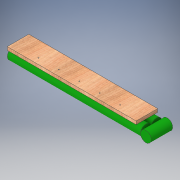
# Autodesk Inventor part: Bumper Side
Saved by Autodesk Inventor 2018 (Build 220112000, 112)
## iProperties
Created: 2019-02-24
Part Number: Bumper Side
Material: Generic
Document SubType Name: Modeling
Designer: maste
Density: 1 g/cm^3
Appearance: Default
Author: maste
Autodesk Inventor part; units mm, degrees
ref_plane "YZ Plane" through (0, 0, 0) normal (1, 0, 0) x (0, 1, 0)
ref_plane "XZ Plane" through (0, 0, 0) normal (0, 1, 0) x (-1, 0, 0)
ref_plane "XY Plane" through (0, 0, 0) normal (0, 0, 1) x (1, 0, 0)
sketch "Sketch1" plane through (0, 0, 0) normal (0, 0, 1) x (1, 0, 0)
  line L0 (0, 0) -> (762, 0)
  line L1 (762, 0) -> (762, 19.05)
  line L2 (762, 19.05) -> (0, 19.05)
  line L3 (0, 19.05) -> (0, 0)
  dimension "d0" = 762
  dimension "d1" = 19.05
  constraints: 8 end point, 2 parallel, 1 horizontal, 1 perpendicular
  measures "d0" distance of L2.end L1.end
  measures "d1" distance of L1.end L0.end
extrude "Extrusion1" add sketch "Sketch1" along normal blind 127
sketch "Sketch2" plane through (0, 0, 0) normal (-1, 0, 0) x (0, 0, 1)
  line L0 (127.1706, 0) -> (127.1706, -31.75) construction
  line L1 (127.1706, -31.75) -> (95.4206, -31.75) construction
  line L2 (95.4206, -31.75) -> (31.9206, -31.75) construction
  circle A0 centre (31.9206, -31.75) radius 31.75
  line L3 (0, 0) -> (127, 0) projected
  circle A1 centre (95.4206, -31.75) radius 31.75
  dimension "d4" = 31.75
  dimension "d5" = 31.75
  dimension "d6" = 63.5
  constraints: 6 end point, 2 centre point, 2 coincident, 2 tangent, 1 perpendicular, 1 point on line, 1 vertical
  measures "d4" distance of L0.start L0.end
  measures "d5" distance of L0.end L1.end
  measures "d6" distance of L1.end L2.end
extrude "Extrusion2" add sketch "Sketch2" against normal blind 787.4 contours A0 | A1
sketch "Sketch4" plane through (0, 0, 127) normal (0, 0, 1) x (1, 0, 0)
  line L0 (0, -31.75) -> (787.4, -31.75) projected
  line L1 (787.4, -31.75) -> (819.15, -31.75) construction
  circle A0 centre (819.15, -31.75) radius 31.75
  point P0 (0, 0)
  dimension "d13" = 31.75
  constraints: 2 end point, 1 coincident, 1 horizontal, 1 horizontal alignment, 2 other
  measures "d13" distance of L0.end L1.end
extrude "Extrusion4" add sketch "Sketch4" against normal blind 127
sketch "Sketch5" plane through (0, 19.05, 0) normal (0, 1, 0) x (1, 0, 0)
  line L0 (0, -127) -> (0, -92.075)
  line L1 (0, 0) -> (0, -127) projected
  line L2 (762, -31.9206) -> (762, -95.4206) construction
  line L3 (0, -92.075) -> (149.225, -92.075) construction
  circle A0 centre (149.225, -92.075) radius 2.5797
  line L4 (149.225, -92.075) -> (269.875, -92.075) construction
  line L5 (269.875, -92.075) -> (390.525, -92.075) construction
  line L6 (390.525, -92.075) -> (511.175, -92.075) construction
  line L7 (511.175, -92.075) -> (631.825, -92.075) construction
  circle A1 centre (269.875, -92.075) radius 2.5797
  circle A2 centre (390.525, -92.075) radius 2.5797
  circle A3 centre (511.175, -92.075) radius 2.5797
  circle A4 centre (631.825, -92.075) radius 2.5797
  dimension "d16" = 34.925
  dimension "d17" = 149.225
  dimension "d30" = 5.1594
  dimension "d33" = 120.65
  dimension "d34" = 120.65
  dimension "d35" = 120.65
  dimension "d36" = 120.65
  constraints: 12 end point, 5 centre point, 5 coincident, 4 point on line, 1 horizontal
  measures "d16" distance of L0.start L0.end
  measures "d17" distance of L0.end L3.end
  measures "d30" diameter of A0
  measures "d33" distance of L4.start L4.end
  measures "d34" distance of L4.end L5.end
  measures "d35" distance of L5.end L6.end
  measures "d36" distance of L6.end L7.end
extrude "Extrusion6" cut sketch "Sketch5" against normal blind 19.05
body "Solid1"
